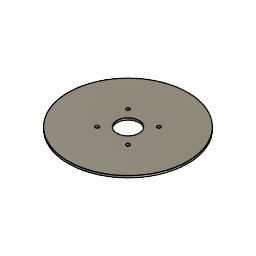
part - base adapter (Autodesk Fusion 360 design; units mm, degrees)
Autodesk Fusion 360 part; units mm, degrees
sketch "Sketch2" plane through (0, 0, 0) normal (0, 0, 1) x (1, 0, 0)
  circle A0 centre (0, 0) radius 60
  line L0 (15.5, 15.5) -> (-15.5, 15.5)
  line L1 (-15.5, 15.5) -> (-15.5, -15.5)
  line L2 (-15.5, -15.5) -> (15.5, -15.5)
  line L3 (15.5, -15.5) -> (15.5, 15.5)
  line L4 (15.5, 15.5) -> (-15.5, -15.5) construction
  line L5 (-15.5, 15.5) -> (15.5, -15.5) construction
  circle A1 centre (-15.5, 15.5) radius 1.7
  circle A2 centre (15.5, 15.5) radius 1.7
  circle A3 centre (-15.5, -15.5) radius 1.7
  circle A4 centre (15.5, -15.5) radius 1.7
  circle A5 centre (0, 0) radius 11.1
  dimension "d2" = 120
  dimension "d8" = 31
  dimension "d9" = 31
  dimension "d10" = 3.4
  dimension "d13" = 31
  dimension "d14" = -31
  dimension "d17" = 22.2
  constraint coincident A0.centre A5.centre
  constraint horizontal L0
  constraint perpendicular L0 L1
  constraint parallel L0 L2
  constraint parallel L1 L3
  constraint coincident L4 A0.centre
  constraint coincident L5 A0.centre
  constraint coincident L0.end L1.start
  measures "d2" diameter of A0
  measures "d8" distance of L0.start L0.end
  measures "d9" distance of L0.end L1.end
  measures "d10" diameter of A1
  measures "d17" diameter of A5
extrude "Extrude2" add sketch "Sketch2" along normal blind 2 contours A0 | L0 L1 L2 L3 A1 A2 A3 A4
convert_to_sheet_metal "ConvertToSheetMetal1"
